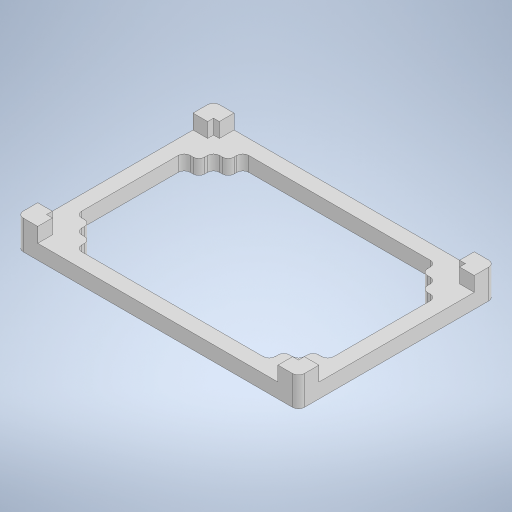
# Autodesk Inventor part: Pi_Case
Saved by Autodesk Inventor 2024 (Build 280153000, 153)
## iProperties
Created: 2024-03-05
Part Number: Pi_Case
Material: 일반
Document SubType Name: Modeling
Designer: SSAFY
Density: 1 g/cm^3
Appearance: 기본값
Author: SSAFY
Autodesk Inventor part; units mm, degrees
ref_plane "YZ Plane" through (0, 0, 0) normal (1, 0, 0) x (0, 1, 0)
ref_plane "XZ Plane" through (0, 0, 0) normal (0, 1, 0) x (-1, 0, 0)
ref_plane "XY Plane" through (0, 0, 0) normal (0, 0, 1) x (1, 0, 0)
sketch "스케치2" plane through (0, 0, 0) normal (0, 1, 0) x (-1, 0, 0)
  line L0 (-43, 28.5) -> (43, 28.5)
  line L1 (43, 28.5) -> (43, -28.5)
  line L2 (43, -28.5) -> (-43, -28.5)
  line L3 (-43, -28.5) -> (-43, 28.5)
  line L4 (-43, 28.5) -> (43, -28.5) construction
  line L5 (43, 28.5) -> (-43, -28.5) construction
  line L6 (-48, -33.5) -> (48, -33.5)
  line L7 (48, -33.5) -> (48, 33.5)
  line L8 (48, 33.5) -> (-48, 33.5)
  line L9 (-48, 33.5) -> (-48, -33.5)
  point P0 (0, 0)
  dimension "d0" = 86
  dimension "d1" = 57
  dimension "d2" = 5
  constraints: 20 end point, 4 parallel, 2 midpoint, 2 perpendicular, 1 horizontal, 3 other
  measures "d0" distance of L1.end L2.end
  measures "d1" distance of L0.end L1.end
  measures "d2" distance between parallel lines of L1 L7
extrude "돌출1" add sketch "스케치2" against normal blind 5 contours L0 L1 L2 L3 | L9 L8 L7 L6
sketch "스케치5" plane through (0, 0, 0) normal (0, 1, 0) x (1, 0, 0)
  line L0 (-48, 33.5) -> (-48, -33.5) projected
  line L1 (-48, -33.5) -> (48, -33.5) projected
  line L2 (48, -33.5) -> (48, 33.5) projected
  line L3 (48, 33.5) -> (-48, 33.5) projected
  line L4 (-43, 28.5) -> (-43, -28.5)
  line L5 (-43, -28.5) -> (43, -28.5)
  line L6 (43, -28.5) -> (43, 28.5)
  line L7 (43, 28.5) -> (-43, 28.5)
  line L8 (-43, 28.5) -> (-33, 28.5)
  line L9 (-33, 28.5) -> (-33, 18.5)
  line L10 (-33, 18.5) -> (-43, 18.5)
  line L11 (-43, 18.5) -> (-43, 28.5)
  line L12 (-33, 18.5) -> (-38, 18.5)
  line L13 (-38, 18.5) -> (-38, 23.5)
  line L14 (-38, 23.5) -> (-33, 23.5)
  line L15 (-33, 23.5) -> (-33, 18.5)
  line L16 (-43, -28.5) -> (-33, -28.5)
  line L17 (-33, -28.5) -> (-33, -18.5)
  line L18 (-33, -18.5) -> (-43, -18.5)
  line L19 (-43, -18.5) -> (-43, -28.5)
  line L20 (-33, -18.5) -> (-38, -18.5)
  line L21 (-38, -18.5) -> (-38, -23.5)
  line L22 (-38, -23.5) -> (-33, -23.5)
  line L23 (-33, -23.5) -> (-33, -18.5)
  line L24 (43, -28.5) -> (33, -28.5)
  line L25 (33, -28.5) -> (33, -18.5)
  line L26 (33, -18.5) -> (43, -18.5)
  line L27 (43, -18.5) -> (43, -28.5)
  line L28 (33, -18.5) -> (38, -18.5)
  line L29 (38, -18.5) -> (38, -23.5)
  line L30 (38, -23.5) -> (33, -23.5)
  line L31 (33, -23.5) -> (33, -18.5)
  line L32 (43, 28.5) -> (33, 28.5)
  line L33 (33, 28.5) -> (33, 18.5)
  line L34 (33, 18.5) -> (43, 18.5)
  line L35 (43, 18.5) -> (43, 28.5)
  line L36 (33, 18.5) -> (38, 18.5)
  line L37 (38, 18.5) -> (38, 23.5)
  line L38 (38, 23.5) -> (33, 23.5)
  line L39 (33, 23.5) -> (33, 18.5)
  point P0 (0, 0)
  dimension "d10" = 5
  dimension "d11" = 10
  dimension "d12" = 10
  dimension "d13" = 5
  dimension "d14" = 5
  dimension "d15" = 10
  dimension "d16" = 10
  dimension "d17" = 5
  dimension "d18" = 5
  dimension "d19" = 10
  dimension "d20" = 10
  dimension "d21" = 5
  dimension "d22" = 5
  dimension "d23" = 10
  dimension "d24" = 10
  dimension "d25" = 5
  dimension "d26" = 5
  constraints: 72 end point, 16 parallel, 8 horizontal, 8 perpendicular, 3 other
  measures "d10" distance between parallel lines of L7 L3
  measures "d11" distance of L9.end L10.end
  measures "d12" distance of L8.end L9.end
  measures "d13" distance of L12.end L13.end
  measures "d14" distance of L13.end L14.end
  measures "d15" distance of L17.end L18.end
  measures "d16" distance of L16.end L17.end
  measures "d17" distance of L20.end L21.end
  measures "d18" distance of L21.end L22.end
  measures "d19" distance of L25.end L26.end
  measures "d20" distance of L24.end L25.end
  measures "d21" distance of L28.end L29.end
  measures "d22" distance of L29.end L30.end
  measures "d23" distance of L32.end L33.end
  measures "d24" distance of L33.end L34.end
  measures "d25" distance of L37.end L38.end
  measures "d26" distance of L36.end L37.end
extrude "돌출3" cut sketch "스케치5" against normal through all contours L10 L9 L7 L33 L34 L6 L26 L25 L5 L17 L18 L4 | L13 L14 L9 L10 | L18 L17 L22 L21 | L38 L37 L34 L33 | L25 L26 L29 L30
sketch "스케치3" plane through (0, 0, 0) normal (0, 1, 0) x (1, 0, 0)
  line L0 (-48, 33.5) -> (-48, -33.5) projected
  line L1 (-48, -33.5) -> (48, -33.5) projected
  line L2 (48, -33.5) -> (48, 33.5) projected
  line L3 (48, 33.5) -> (-48, 33.5) projected
  line L4 (-43, 28.5) -> (-43, -28.5)
  line L5 (-43, -28.5) -> (43, -28.5)
  line L6 (43, -28.5) -> (43, 28.5)
  line L7 (43, 28.5) -> (-43, 28.5)
  line L8 (-48, 26.5) -> (-43, 26.5)
  line L9 (-41, 33.5) -> (-41, 28.5)
  point P0 (0, 0)
  dimension "d5" = 5
  dimension "d6" = 7
  dimension "d7" = 7
  constraints: 12 end point, 4 point on line, 2 perpendicular, 3 other
  measures "d5" distance between parallel lines of L4 L0
  measures "d6" distance between parallel lines of L9 L0
  measures "d7" distance between parallel lines of L3 L8
extrude "돌출2" add sketch "스케치3" along normal blind 5 contours L3 L9 L7 L4 L8 L0
mirror "미러1" about plane through (0, 0, 0) normal (1, 0, 0) of "돌출2"
mirror "미러2" about plane through (0, 0, 0) normal (0, 0, 1) of "돌출2", "미러1"
fillet "모깎기1" radius 2 24 edges at (-33, -2.5, 28.5) (-33, -2.5, 23.5) (-38, -2.5, 23.5) (-38, -2.5, 18.5) (-43, -2.5, 18.5) (-48, 0, 33.5) (-48, 0, -33.5) (48, 0, -33.5) (48, 0, 33.5) (-43, -2.5, -18.5) (-38, -2.5, -18.5) (-38, -2.5, -23.5) (-33, -2.5, -23.5) (-33, -2.5, -28.5) (33, -2.5, -28.5) (33, -2.5, -23.5) (38, -2.5, -23.5) (38, -2.5, -18.5) (43, -2.5, -18.5) (43, -2.5, 18.5) (38, -2.5, 18.5) (38, -2.5, 23.5) (33, -2.5, 23.5) (33, -2.5, 28.5)
